Autodesk Inventor part; units mm, degrees
(part 2 of 2)
sketch "Sketch27" plane through (6.5069, 0, -114.9941) normal (1, 0, 0) x (0, 0, -1)
  line L0 (1.4806, -10) -> (-8.5181, -10) projected
  line L1 (-18.5231, 0) -> (-18.5231, 5) projected
  line L2 (-8.5181, -10) -> (-18.5231, 0)
  line L3 (-18.5231, 0) -> (-8.5181, 0)
  line L4 (-6.9885, 5) -> (-6.9885, -10) projected
  line L5 (-8.5181, 0) -> (-8.5181, -10)
  point P0 (-114.9941, 0)
  constraints: 6 end point, 2 perpendicular
extrude "Extrusion31" add sketch "Sketch27" against normal blind 3
sketch "Sketch28" plane through (-29.9992, 0, -101.4702) normal (0, 0, 1) x (1, 0, 0)
  line L0 (0, 0) -> (0, 4) projected
  line L1 (0, 0) -> (17.8885, -30.9838)
  line L2 (5, 0) -> (0, 0)
  line L3 (-0.5001, 0) -> (-0.5001, 5) projected
  line L4 (10.9985, 0) -> (11.1697, -10.6862)
  line L5 (7.9991, 0) -> (7.9991, 5) projected
  line L6 (59.9982, 0) -> (42.1012, -30.9838)
  line L7 (54.9911, 0) -> (59.9982, 0)
  line L8 (22.9431, -25.9835) -> (20.0017, -25.9838)
  line L9 (22.9431, -25.9835) -> (40.0425, -25.9819)
  line L10 (51.9997, 0) -> (51.9997, -5.1787)
  line L11 (48.9997, 0) -> (48.9997, -10.475)
  line L12 (40.0425, -25.9819) -> (48.9997, -10.475)
  line L13 (51.9997, -5.1787) -> (54.9911, 0)
  line L14 (20.0017, -25.9838) -> (11.1697, -10.6862)
  line L15 (7.9991, -5.1946) -> (5, 0)
  line L16 (17.8885, -30.9838) -> (42.1012, -30.9838)
  line L17 (48.9997, 0) -> (51.9997, 0)
  line L18 (52.0003, 5) -> (7.9991, 5) projected
  line L19 (10.9985, 0) -> (7.9985, 0)
  line L20 (7.9985, 0) -> (7.9985, -5.1935)
  point P0 (29.9992, 0)
  constraints: 34 end point, 6 parallel, 5 point on line, 2 vertical, 1 horizontal, 1 perpendicular
extrude "Extrusion32" add sketch "Sketch28" against normal blind 5
sketch "Sketch29" plane through (-12.1107, -30.9838, -101.4702) normal (0, -1, 0) x (1, 0, 0)
  circle A0 centre (12.1, -2.5) radius 1.75
  point P0 (12.1107, 101.4702)
  constraints: 1 centre point
sketch "Sketch30" plane through (-12.1107, -30.9838, -101.4702) normal (0, -1, 0) x (1, 0, 0)
  line L0 (17.1, -7.5) -> (7.1, -7.5)
  line L1 (7.1, -7.5) -> (7.1, 2.5)
  line L2 (7.1, 2.5) -> (17.1, 2.5)
  line L3 (17.1, 2.5) -> (17.1, -7.5)
  line L4 (17.1, -7.5) -> (7.1, 2.5) construction
  line L5 (7.1, -7.5) -> (17.1, 2.5) construction
  circle A0 centre (12.1, -2.5) radius 1.75
  point P0 (12.1107, 101.4702)
  constraints: 12 end point, 2 midpoint, 2 parallel, 1 centre point, 1 coincident, 1 horizontal, 1 perpendicular
extrude "Extrusion34" add sketch "Sketch30" against normal blind 5
extrude "Extrusion35" cut sketch "Sketch29" against normal blind 6
sketch "Sketch31" plane through (12.1019, -30.9838, -106.4702) normal (0, -1, 0) x (1, 0, 0)
  line L0 (-17.1127, 5) -> (-17.1127, 7.5) projected
  line L1 (-7.1127, 7.5) -> (-7.1127, 5) projected
  line L2 (-17.1127, 7.5) -> (-7.1127, 7.5)
  line L3 (-7.1127, 7.5) -> (-7.1127, 6.25)
  line L4 (-7.1127, 6.25) -> (-17.1127, 6.25)
  line L5 (-17.1127, 6.25) -> (-17.1127, 7.5)
  point P0 (-12.1019, 106.4702)
  constraints: 8 end point, 2 parallel, 1 horizontal, 1 midpoint, 1 perpendicular
extrude "Extrusion36" cut sketch "Sketch31" against normal blind 6
sketch "Sketch32" plane through (-12.1107, -30.9838, -106.4702) normal (0, -1, 0) x (1, 0, 0)
  line L0 (7.1, 6.25) -> (17.1, 6.25) projected
  line L1 (17.1, 6.25) -> (17.1, 5) projected
  line L2 (7.1, 6.25) -> (17.1, 6.25)
  line L3 (17.1, 6.25) -> (17.1, 5.75)
  line L4 (17.1, 5.75) -> (7.1, 5.75)
  line L5 (7.1, 5.75) -> (7.1, 6.25)
  line L6 (17.1, -2.5) -> (7.1, -2.5) projected
  line L7 (17.1, 0) -> (17.1, -2.5) projected
  line L8 (7.1, -2.5) -> (17.1, -2.5)
  line L9 (17.1, -2.5) -> (17.1, -0.75)
  line L10 (17.1, -0.75) -> (7.1, -0.75)
  line L11 (7.1, -0.75) -> (7.1, -2.5)
  point P0 (12.1107, 106.4702)
  dimension "d218" = 0.5
  dimension "d219" = 1.75
  constraints: 16 end point, 4 parallel, 2 horizontal, 2 perpendicular, 2 point on line
  measures "d218" distance of L2.end L3.end
  measures "d219" distance of L9.end L8.end
extrude "Extrusion37" cut sketch "Sketch32" against normal blind 6
sketch "Sketch33" plane through (0, 0, 0) normal (0, -1, 0) x (1, 0, 0)
  circle A0 centre (-23.9996, -27) radius 1.5 projected
  circle A1 centre (-23.9996, -27) radius 1.75
  circle A2 centre (-23.9996, -82.9885) radius 1.75
  circle A3 centre (23.9996, -83) radius 1.5 projected
  circle A4 centre (23.9996, -83) radius 1.75
  circle A5 centre (23.9996, -27) radius 1.75
  circle A6 centre (30.4217, -15.0386) radius 1.1 projected
  circle A7 centre (30.4217, -15.0386) radius 1.25
  circle A8 centre (39.4723, -5.9876) radius 2 projected
  circle A9 centre (39.4723, -5.9876) radius 1.25
  circle A10 centre (-30.4214, -15.0386) radius 1.1 projected
  circle A11 centre (-30.4214, -15.0386) radius 1.25
  circle A12 centre (-39.4723, -5.9876) radius 1.1 projected
  circle A13 centre (-39.4723, -5.9876) radius 1.25
  point P0 (0, 0)
  dimension "d222" = 3.5
  dimension "d223" = 3.5
  dimension "d224" = 3.5
  dimension "d225" = 3.5
  dimension "d226" = 2.5
  dimension "d227" = 2.5
  dimension "d228" = 2.5
  dimension "d229" = 2.5
  constraints: 8 centre point, 6 coincident
  measures "d222" diameter of A1
  measures "d223" diameter of A2
  measures "d224" diameter of A4
  measures "d225" diameter of A5
  measures "d226" diameter of A7
  measures "d227" diameter of A9
  measures "d228" diameter of A11
  measures "d229" diameter of A13
extrude "Extrusion38" cut sketch "Sketch33" against normal blind 6 contours A1 | A2 | A4 | A5 | A7 | A9 | A11 | A13
sketch "Sketch34" plane through (0, 4, 0) normal (0, -1, 0) x (1, 0, 0)
  line L0 (-37.7403, -29.9253) -> (-18.1375, -29.9253) construction
  line L1 (-18.1375, -29.9253) -> (-18.1375, -37.5548) construction
  line L2 (-18.1375, -37.5548) -> (-37.7403, -37.5548) construction
  line L3 (-37.7403, -37.5548) -> (-37.7403, -29.9253) construction
  line L4 (-31.8924, -36.0253) -> (-32.7031, -36.0253)
  line L5 (-32.7031, -36.0253) -> (-32.7031, -30.7706)
  line L6 (-32.7031, -30.7706) -> (-34.2948, -34.3446)
  line L7 (-34.2948, -34.3446) -> (-34.7892, -34.3446)
  line L8 (-34.7892, -34.3446) -> (-36.3661, -30.7706)
  line L9 (-36.3661, -30.7706) -> (-36.3661, -36.0253)
  line L10 (-36.3661, -36.0253) -> (-37.1224, -36.0253)
  line L11 (-37.1224, -36.0253) -> (-37.1224, -29.9253)
  line L12 (-37.1224, -29.9253) -> (-36.0151, -29.9253)
  line L13 (-36.0151, -29.9253) -> (-34.4926, -33.3213)
  line L14 (-34.4926, -33.3213) -> (-33.0195, -29.9253)
  line L15 (-33.0195, -29.9253) -> (-31.8924, -29.9253)
  line L16 (-31.8924, -29.9253) -> (-31.8924, -36.0253)
  line L17 (-26.2076, -36.0253) -> (-27.2606, -36.0253)
  line L18 (-27.2606, -36.0253) -> (-29.49, -33.1879)
  line L19 (-29.49, -33.1879) -> (-29.8459, -33.5883)
  line L20 (-29.8459, -33.5883) -> (-29.8459, -36.0253)
  line L21 (-29.8459, -36.0253) -> (-30.6566, -36.0253)
  line L22 (-30.6566, -36.0253) -> (-30.6566, -29.9253)
  line L23 (-30.6566, -29.9253) -> (-29.8459, -29.9253)
  line L24 (-29.8459, -29.9253) -> (-29.8459, -32.7281)
  line L25 (-29.8459, -32.7281) -> (-27.3446, -29.9253)
  line L26 (-27.3446, -29.9253) -> (-26.3559, -29.9253)
  line L27 (-26.3559, -29.9253) -> (-28.882, -32.6491)
  line L28 (-28.882, -32.6491) -> (-26.2076, -36.0253)
  line L29 (-19.4452, -30.8398) -> (-22.085, -36.0253)
  line L30 (-22.085, -36.0253) -> (-22.955, -36.0253)
  line L31 (-22.955, -36.0253) -> (-20.167, -30.6421)
  line L32 (-20.167, -30.6421) -> (-23.3158, -30.6421)
  line L33 (-23.3158, -30.6421) -> (-23.3158, -29.9253)
  line L34 (-23.3158, -29.9253) -> (-19.4452, -29.9253)
  line L35 (-19.4452, -29.9253) -> (-19.4452, -30.8398)
  point P0 (0, 0)
  constraints: 2 other
extrude "Extrusion39" add sketch "Sketch34" along normal blind 2
body "Solid4"
